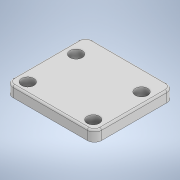
# Autodesk Inventor part: cylinder head
Saved by Autodesk Inventor 2020 (Build 240168000, 168)
## iProperties
Created: 2020-08-05
Part Number: cylinder head
Material: Generic
Document SubType Name: Modeling
Designer: benny
Density: 1 g/cm^3
Appearance: Default
Author: benny
Autodesk Inventor part; units mm, degrees
ref_plane "YZ Plane" through (0, 0, 0) normal (1, 0, 0) x (0, 1, 0)
ref_plane "XZ Plane" through (0, 0, 0) normal (0, 1, 0) x (-1, 0, 0)
ref_plane "XY Plane" through (0, 0, 0) normal (0, 0, 1) x (1, 0, 0)
sketch "Sketch1" plane through (0, 0, 0) normal (0, 1, 0) x (-1, 0, 0)
  line L0 (25, -25.5) -> (-25, -25.5)
  line L1 (-25, -25.5) -> (-25, 19.5)
  line L2 (-25, 19.5) -> (25, 19.5)
  line L3 (25, 19.5) -> (25, -25.5)
  line L4 (25, -25.5) -> (-25, 19.5) construction
  line L5 (-25, -25.5) -> (25, 19.5) construction
  point P0 (0, 0)
  point P1 (0, -3)
  dimension "d0" = 50
  dimension "d1" = 45
  constraints: 12 end point, 2 midpoint, 2 parallel, 1 horizontal, 1 perpendicular
  measures "d0" distance of L1.end L2.end
  measures "d1" distance of L0.end L1.end
extrude "Extrusion1" add sketch "Sketch1" along normal blind 6
fillet "Fillet1" radius 4 4 edges at (25, 3, 19.5) (25, 3, -25.5) (-25, 3, -25.5) (-25, 3, 19.5)
fillet "Fillet2" radius 1 8 edges at (23.8284, 6, 18.3284) (25, 6, -3) (23.8284, 6, -24.3284) (0, 6, -25.5) (-23.8284, 6, -24.3284) (-25, 6, -3) (-23.8284, 6, 18.3284) (0, 6, 19.5)
sketch "Sketch3" plane through (0, 6, 0) normal (0, 1, 0) x (1, 0, 0)
  line L0 (0, 0) -> (-18.5052, -13.6586)
  circle A0 centre (-18.5052, -13.6586) radius 3.5
  dimension "d11" = 23
  dimension "d12" = 7
  constraints: 2 end point, 1 centre point, 1 coincident
  measures "d11" distance of L0.start L0.end
  measures "d12" diameter of A0
extrude "Extrusion3" cut sketch "Sketch3" against normal blind 6
mirror "Mirror1" about plane through (0, 0, 0) normal (1, 0, 0) of "Extrusion3"
mirror "Mirror2" about plane through (0, 0, 0) normal (0, 0, 1) of "Extrusion3", "Mirror1"
body "Solid1"
